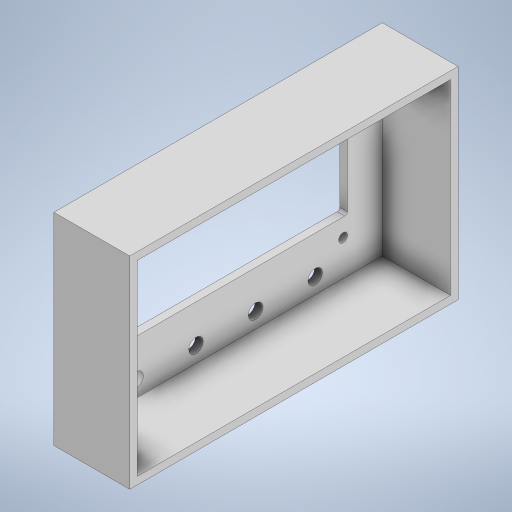
# Autodesk Inventor part: cover lcd
Saved by Autodesk Inventor 2023 (Build 270158030, 158C)
## iProperties
Created: 2023-03-06
Part Number: cover lcd
Material: Generic
Document SubType Name: Modeling
Designer: fatih
Density: 1 g/cm^3
Appearance: Default
Author: fatih
Autodesk Inventor part; units mm, degrees
ref_plane "YZ Plane" through (0, 0, 0) normal (1, 0, 0) x (0, 1, 0)
ref_plane "XZ Plane" through (0, 0, 0) normal (0, 1, 0) x (-1, 0, 0)
ref_plane "XY Plane" through (0, 0, 0) normal (0, 0, 1) x (1, 0, 0)
sketch "Sketch1" plane through (0, 0, 0) normal (1, 0, 0) x (0, 1, 0)
  line L0 (0, 0) -> (80, 0)
  line L1 (80, 0) -> (80, -130)
  line L2 (80, -130) -> (0, -130)
  line L3 (0, -130) -> (0, 0)
  dimension "d0" = 130
  dimension "d1" = 80
  constraints: 8 end point, 2 parallel, 1 horizontal, 1 perpendicular
  measures "d0" distance of L0.end L1.end
  measures "d1" distance of L0.start L0.end
extrude "Extrusion1" add sketch "Sketch1" along normal blind 30
shell "Shell1" thickness 3 removed faces 1 at (30, 53.3333, -43.3333)
sketch "Sketch2" plane through (0, 0, 0) normal (-1, 0, 0) x (0, 0, 1)
  line L0 (-127, 77) -> (-3, 77) projected
  line L1 (-127, 3) -> (-3, 3) projected
  line L2 (-127, 77) -> (-3, 77)
  line L3 (-3, 77) -> (-3, 3)
  line L4 (-3, 3) -> (-127, 3)
  line L5 (-127, 3) -> (-127, 77)
  line L6 (-65, 77) -> (-65, 41.725)
  line L7 (-127, 77) -> (-122, 77)
  line L8 (-122, 77) -> (-122, 72)
  line L9 (-122, 72) -> (-127, 72)
  line L10 (-127, 72) -> (-127, 77)
  line L11 (-3, 77) -> (-8, 77)
  line L12 (-8, 77) -> (-8, 72)
  line L13 (-8, 72) -> (-3, 72)
  line L14 (-3, 72) -> (-3, 77)
  circle A0 centre (-18.54, 72) radius 1.75
  circle A1 centre (-111.46, 72) radius 1.75
  line L15 (-111.46, 17.08) -> (-18.54, 17.08)
  circle A2 centre (-111.46, 17.08) radius 1.75
  circle A3 centre (-18.54, 17.08) radius 1.75
  line L16 (-111.46, 72) -> (-111.46, 64.54)
  line L17 (-65, 64.54) -> (-16.8, 64.54)
  line L18 (-17.8, 64.54) -> (-112.2, 64.54)
  line L19 (-113.2, 63.54) -> (-113.2, 25.14)
  line L20 (-112.2, 24.14) -> (-17.8, 24.14)
  line L21 (-16.8, 25.14) -> (-16.8, 63.54)
  arc A4 (-112.2, 64.54) -> (-113.2, 63.54) centre (-112.2, 63.54) ccw
  arc A5 (-113.2, 25.14) -> (-112.2, 24.14) centre (-112.2, 25.14) ccw
  arc A6 (-17.8, 24.14) -> (-16.8, 25.14) centre (-17.8, 25.14) ccw
  arc A7 (-16.8, 63.54) -> (-17.8, 64.54) centre (-17.8, 63.54) ccw
  point P0 (0, 0)
  point P1 (-113.2, 64.54)
  point P2 (-113.2, 24.14)
  dimension "d5" = 5
  dimension "d6" = 5
  dimension "d7" = 5
  dimension "d8" = 5
  dimension "d11" = 3.5
  dimension "d12" = 3.5
  dimension "d13" = 54.92
  dimension "d14" = 3.5
  dimension "d15" = 3.5
  dimension "d16" = 7.46
  dimension "d18" = 92.92
  dimension "d19" = 48.2
  dimension "d20" = 96.4
  dimension "d21" = 40.4
  dimension "d22" = 1
  constraints: 40 end point, 8 centre point, 8 point on circle, 8 point on line, 8 tangent, 6 parallel, 5 perpendicular, 4 horizontal, 3 equal radius, 3 vertical, 2 coincident, 1 midpoint
  measures "d5" distance of L8.end L9.end
  measures "d6" distance of L7.end L8.end
  measures "d7" distance of L13.end L12.end
  measures "d8" distance of L12.end L11.end
  measures "d11" diameter of A0
  measures "d12" diameter of A1
  measures "d13" distance of L16.start L15.start
  measures "d14" diameter of A2
  measures "d15" diameter of A3
  measures "d16" distance of L16.start L16.end
  measures "d18" distance of A0.centre L16.start
  measures "d19" distance of L17.start L17.end
  measures "d20" distance of L17.end point (-113.2, 64.54)
  measures "d21" distance of point (-113.2, 64.54) point (-113.2, 24.14)
  measures "d22" radius of A4
extrude "Extrusion2" cut sketch "Sketch2" against normal blind 30 contours A0 | A1 | A2 | A3 | L17 A7 L21 A6 L20 A5 L19 A4 L18
sketch "Sketch3" plane through (0, 0, 0) normal (-1, 0, 0) x (0, 0, 1)
  line L0 (-17.8, 24.14) -> (-112.2, 24.14) projected
  line L1 (-65, 24.14) -> (-65, 0)
  line L2 (0, 0) -> (-130, 0) projected
  line L3 (-65, 9.22) -> (-65, 12.07)
  line L4 (-65, 10.645) -> (-64.0682, 10.645)
  circle A0 centre (-53.2, 9.22) radius 2.85
  circle A1 centre (-29.6, 9.22) radius 2.85
  circle A2 centre (-76.8, 9.22) radius 2.85
  circle A3 centre (-100.4, 9.22) radius 2.85
  line L5 (-65, 12.07) -> (-65, 9.22)
  point P0 (-88.6, 12.07)
  point P1 (-88.6, 9.22)
  constraints: 8 end point, 4 centre point, 4 midpoint, 3 symmetric about line, 1 horizontal, 1 point on line
extrude "Extrusion3" cut sketch "Sketch3" against normal blind 30
body "Solid1"
